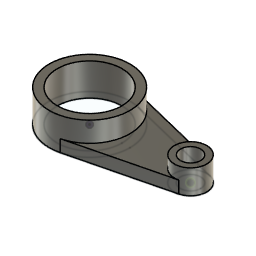
6주 예제 1 (Autodesk Fusion 360 design; units mm, degrees)
Autodesk Fusion 360 part; units mm, degrees
sketch "스케치1" plane through (0, 0, 0) normal (0, 0, 1) x (1, 0, 0)
  circle A0 centre (0, 0) radius 50
  circle A1 centre (125.1784, 0) radius 20
  line L0 (11.9829, 48.5429) -> (129.9716, 19.4171)
  line L1 (11.9829, -48.5429) -> (129.9716, -19.4171)
  circle A2 centre (0, 0) radius 40
  circle A3 centre (125.1784, 0) radius 12.5
  dimension "d1" = 100
  dimension "d2" = 40
  dimension "d3" = 80
  dimension "d4" = 25
  constraint coincident A0.centre A2.centre
  constraint coincident A0 L0.start
  constraint coincident A1 L0.end
  constraint tangent A1 L0
  constraint coincident A0 L1.start
  constraint coincident A1 L1.end
  constraint tangent A1 L1
  constraint tangent A0 L0
  constraint tangent A0 L1
  constraint concentric A1 A3
  measures "d1" diameter of A0
  measures "d2" diameter of A1
  measures "d3" diameter of A2
  measures "d4" diameter of A3
extrude "돌출4" add sketch "스케치1" along normal blind 40 contours A0 makes body 1
extrude "돌출5" add sketch "스케치1" along normal blind 30 separate body contours A1 makes body 2
extrude "돌출6" add sketch "스케치1" along normal blind 15 contours A0 A1 L0 L1 bodies 1 2
